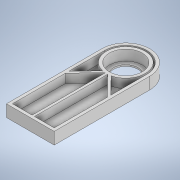
# Autodesk Inventor part: FlanecPodsipnikForwardBabka
Saved by Autodesk Inventor 2022 (Build 260153000, 153)
## iProperties
Created: 2023-08-16
Part Number: FlanecPodsipnikForwardBabka
Material: Generic
Document SubType Name: Modeling
Designer: Kippi
Density: 1 g/cm^3
Appearance: Default
Author: Kippi
Autodesk Inventor part; units mm, degrees
ref_plane "YZ Plane" through (0, 0, 0) normal (1, 0, 0) x (0, 1, 0)
ref_plane "XZ Plane" through (0, 0, 0) normal (0, 1, 0) x (-1, 0, 0)
ref_plane "XY Plane" through (0, 0, 0) normal (0, 0, 1) x (1, 0, 0)
sketch "Sketch1" plane through (0, 0, 0) normal (0, 1, 0) x (-1, 0, 0)
  line L0 (64, 229.3333) -> (-96, 229.3333)
  line L1 (-96, 229.3333) -> (-96, -170.6667)
  line L2 (-96, -170.6667) -> (64, -170.6667)
  line L3 (64, -170.6667) -> (64, 229.3333)
  circle A0 centre (-16, -90.6667) radius 80
  circle A1 centre (-16, -90.6667) radius 40
  circle A2 centre (-16, -90.6667) radius 55
  point P0 (0, 0)
  point P1 (-96, -90.6667)
  point P2 (64, -90.6667)
  dimension "d0" = 160
  dimension "d1" = 400
  dimension "d2" = 80
  dimension "d3" = 110
  constraints: 8 end point, 3 centre point, 3 tangent, 2 coincident, 2 parallel, 1 horizontal, 1 perpendicular
  measures "d0" distance of L1.end L2.end
  measures "d1" distance of L2.end L0.start
  measures "d2" diameter of A1
  measures "d3" diameter of A2
extrude "Extrusion1" add sketch "Sketch1" along normal blind 40 contours L3 A0 L1 L0 | A0
sketch "Sketch2" plane through (0, 0, 0) normal (0, -1, 0) x (1, 0, 0)
  circle A0 centre (16, -90.6667) radius 55 construction
  circle A1 centre (16, -90.6667) radius 40.5
  circle A2 centre (16, -90.6667) radius 55
  point P0 (0, 0)
  dimension "d14" = 81
  constraints: 2 centre point, 2 coincident, 1 concentric
  measures "d14" diameter of A1
extrude "Extrusion2" add sketch "Sketch2" against normal blind 5
sketch "Sketch3" plane through (0, 40, 0) normal (0, 1, 0) x (1, 0, 0)
  line L0 (-64, 90.6667) -> (-64, -229.3333) construction
  line L1 (-64, -229.3333) -> (96, -229.3333) construction
  line L2 (96, -229.3333) -> (96, 90.6667) construction
  arc A0 (96, 90.6667) -> (-64, 90.6667) centre (16, 90.6667) ccw construction
  circle A1 centre (16, 90.6667) radius 55 construction
  line L3 (-64, 90.6667) -> (-64, -229.3333) construction
  line L4 (-64, -229.3333) -> (96, -229.3333) construction
  line L5 (96, -229.3333) -> (96, 90.6667) construction
  arc A2 (96, 90.6667) -> (-64, 90.6667) centre (16, 90.6667) ccw construction
  circle A3 centre (16, 90.6667) radius 55 construction
  line L6 (-54, -219.3333) -> (-54, 90.6667)
  arc A4 (86, 90.6667) -> (-54, 90.6667) centre (16, 90.6667) ccw
  line L7 (86, 90.6667) -> (86, -219.3333)
  line L8 (86, -219.3333) -> (-54, -219.3333)
  circle A5 centre (16, 90.6667) radius 65
  line L9 (12, 31.7512) -> (20, 31.7512)
  line L10 (20, 31.7512) -> (20, -221.1661)
  line L11 (20, -221.1661) -> (12, -221.1661)
  line L12 (12, -221.1661) -> (12, 31.7512)
  line L13 (12, 26) -> (-54, -41)
  line L14 (20, 26) -> (86, -41)
  line L15 (6.3008, 31.6142) -> (-59.6992, -35.3858)
  line L16 (25.6992, 31.6142) -> (91.6992, -35.3858)
  point P0 (0, 0)
  point P1 (20.1949, 25.8022)
  point P2 (20, 25.7899)
  point P3 (20, -219.3333)
  point P4 (11.8051, 25.8022)
  point P5 (12, -219.3333)
  point P6 (12, 25.7899)
  point P7 (-54, -29.6003)
  point P8 (1.9547, 27.2023)
  point P9 (30.0453, 27.2023)
  point P10 (86, -29.6003)
  dimension "d8" = 10
  dimension "d9" = 10
  dimension "d10" = 8
  dimension "d11" = 8
  constraints: 22 end point, 4 parallel, 4 point on line, 2 centre point, 2 point on circle, 1 horizontal, 1 perpendicular, 3 other
  measures "d8" radial gap between concentric circles of A5 A1
  measures "d9" distance between parallel lines of L0 L6
  measures "d10" distance between parallel lines of L14 L16
  measures "d11" distance between parallel lines of L13 L15
extrude "Extrusion3" cut sketch "Sketch3" against normal blind 30 contours L6 L13 A5 L12 L8 | L6 A4 L7 L16 A5 L15 | L10 A5 L14 L7 L8
body "Solid1"
